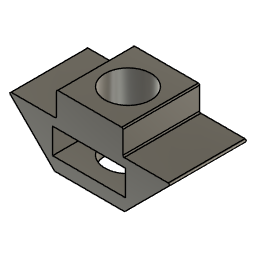
t-slot-nut (Autodesk Fusion 360 design; units mm, degrees)
Autodesk Fusion 360 part; units mm, degrees
sketch "Sketch1" plane through (0, 0, 0) normal (0, 1, 0) x (1, 0, 0) in component "2020-extrusion v1"
  line L0 (9, -10) -> (-9, -10)
  line L1 (-10, -9) -> (-10, 9)
  line L2 (-9, 10) -> (9, 10)
  line L3 (10, 9) -> (10, -9)
  line L4 (10, -10) -> (-10, 10) construction
  line L5 (-10, -10) -> (10, 10) construction
  line L6 (4, -4) -> (-4, -4)
  line L7 (-4, -4) -> (-4, 4)
  line L8 (-4, 4) -> (4, 4)
  line L9 (4, 4) -> (4, -4)
  line L10 (4, -4) -> (-4, 4) construction
  line L11 (-4, -4) -> (4, 4) construction
  circle A0 centre (0, 0) radius 2
  line L12 (8.45, -8.45) -> (-8.45, -8.45)
  line L13 (-8.45, -8.45) -> (-8.45, 8.45)
  line L14 (-8.45, 8.45) -> (8.45, 8.45)
  line L15 (8.45, 8.45) -> (8.45, -8.45)
  line L16 (8.45, -8.45) -> (-8.45, 8.45) construction
  line L17 (-8.45, -8.45) -> (8.45, 8.45) construction
  line L18 (-9.452, -10.548) -> (10.548, 9.452) construction
  line L19 (-10.548, -9.452) -> (9.452, 10.548) construction
  line L20 (10.548, -9.452) -> (-9.452, 10.548) construction
  line L21 (9.452, -10.548) -> (-10.548, 9.452) construction
  line L22 (3.1, -10) -> (-3.1, -10) construction
  line L23 (-3.1, -10) -> (-3.1, 10) construction
  line L24 (-3.1, 10) -> (3.1, 10) construction
  line L25 (3.1, 10) -> (3.1, -10) construction
  line L26 (10, -3.1) -> (-10, -3.1) construction
  line L27 (-10, -3.1) -> (-10, 3.1) construction
  line L28 (-10, 3.1) -> (10, 3.1) construction
  line L29 (10, 3.1) -> (10, -3.1) construction
  line L30 (-3.1, -8.45) -> (-3.1, -10)
  line L31 (3.1, -8.45) -> (3.1, -10)
  line L32 (-8.45, -3.1) -> (-10, -3.1)
  line L33 (-8.45, 3.1) -> (-10, 3.1)
  line L34 (8.45, -3.1) -> (10, -3.1)
  line L35 (8.45, 3.1) -> (10, 3.1)
  line L36 (-3.1, 8.45) -> (-3.1, 10)
  line L37 (3.1, 8.45) -> (3.1, 10)
  line L38 (-4, 2.904) -> (-8.45, 7.354)
  line L39 (-2.904, 4) -> (-7.354, 8.45)
  line L40 (2.904, 4) -> (7.354, 8.45)
  line L41 (4, 2.904) -> (8.45, 7.354)
  line L42 (-4, -2.904) -> (-8.45, -7.354)
  line L43 (-2.904, -4) -> (-7.354, -8.45)
  line L44 (2.904, -4) -> (7.354, -8.45)
  line L45 (4, -2.904) -> (8.45, -7.354)
  line L46 (-10, -3.1) -> (-9.55, -3.1)
  line L47 (-9.55, -3.1) -> (-9.55, -3.6)
  line L48 (-9.55, -3.6) -> (-10, -3.6)
  line L49 (-10, -3.6) -> (-10, -3.1)
  line L50 (-10, 3.1) -> (-9.55, 3.1)
  line L51 (-9.55, 3.1) -> (-9.55, 3.6)
  line L52 (-9.55, 3.6) -> (-10, 3.6)
  line L53 (-10, 3.6) -> (-10, 3.1)
  line L54 (-3.1, -10) -> (-3.6, -10)
  line L55 (-3.6, -10) -> (-3.6, -9.55)
  line L56 (-3.6, -9.55) -> (-3.1, -9.55)
  line L57 (-3.1, -9.55) -> (-3.1, -10)
  line L58 (3.1, -10) -> (3.6, -10)
  line L59 (3.6, -10) -> (3.6, -9.55)
  line L60 (3.6, -9.55) -> (3.1, -9.55)
  line L61 (3.1, -9.55) -> (3.1, -10)
  line L62 (10, -3.1) -> (9.55, -3.1)
  line L63 (9.55, -3.1) -> (9.55, -3.6)
  line L64 (9.55, -3.6) -> (10, -3.6)
  line L65 (10, -3.6) -> (10, -3.1)
  line L66 (10, 3.1) -> (9.55, 3.1)
  line L67 (9.55, 3.1) -> (9.55, 3.6)
  line L68 (9.55, 3.6) -> (10, 3.6)
  line L69 (10, 3.6) -> (10, 3.1)
  line L70 (-3.1, 10) -> (-3.6, 10)
  line L71 (-3.6, 10) -> (-3.6, 9.55)
  line L72 (-3.6, 9.55) -> (-3.1, 9.55)
  line L73 (-3.1, 9.55) -> (-3.1, 10)
  line L74 (3.1, 10) -> (3.55, 10)
  line L75 (3.55, 10) -> (3.55, 9.5)
  line L76 (3.55, 9.5) -> (3.1, 9.5)
  line L77 (3.1, 9.5) -> (3.1, 10)
  arc A1 (-10, -9) -> (-9, -10) centre (-9, -9) ccw
  arc A2 (9, -10) -> (10, -9) centre (9, -9) ccw
  arc A3 (10, 9) -> (9, 10) centre (9, 9) ccw
  arc A4 (-9, 10) -> (-10, 9) centre (-9, 9) ccw
  dimension "d1" = 20
  dimension "d2" = 20
  dimension "d3" = 8
  dimension "d4" = 8
  dimension "d5" = 4
  dimension "d6" = 16.9
  dimension "d7" = 16.9
  dimension "d8" = 0.775
  dimension "d9" = -0.775
  dimension "d10" = 0.775
  dimension "d11" = -0.775
  dimension "d12" = 6.2
  dimension "d13" = 20
  dimension "d14" = 20
  dimension "d15" = 6.2
  dimension "d16" = 1.55
  dimension "d17" = 1.55
  dimension "d18" = 1.55
  dimension "d19" = 1.55
  dimension "d20" = 1.55
  dimension "d21" = 1.55
  dimension "d22" = 1.55
  dimension "d23" = 1.55
  dimension "d24" = 0.45
  dimension "d25" = 0.5
  dimension "d26" = 0.45
  dimension "d27" = 0.5
  dimension "d28" = 0.5
  dimension "d29" = 0.45
  dimension "d30" = 0.5
  dimension "d31" = 0.45
  dimension "d32" = 0.45
  dimension "d33" = 0.5
  dimension "d34" = 0.45
  dimension "d35" = 0.5
  dimension "d36" = 0.5
  dimension "d37" = 0.45
  dimension "d38" = 0.45
  dimension "d39" = 0.5
  dimension "d40" = 1
  dimension "d41" = 1
  dimension "d42" = 1
  dimension "d43" = 1
  constraint horizontal L0
  constraint perpendicular L0 L1
  constraint parallel L0 L2
  constraint parallel L1 L3
  constraint coincident L4 A0.centre
  constraint coincident L5 A0.centre
  constraint coincident A0.centre origin
  constraint horizontal L6
  constraint perpendicular L6 L7
  constraint parallel L6 L8
  constraint parallel L7 L9
  constraint coincident L10 A0.centre
  constraint coincident L11 A0.centre
  constraint horizontal L12
  constraint perpendicular L12 L13
  constraint parallel L12 L14
  constraint parallel L13 L15
  constraint coincident L16 A0.centre
  constraint coincident L17 A0.centre
  constraint horizontal L22
  constraint perpendicular L22 L23
  constraint parallel L22 L24
  constraint parallel L23 L25
  constraint horizontal L26
  constraint perpendicular L26 L27
  constraint parallel L26 L28
  constraint parallel L27 L29
  constraint vertical L30
  constraint coincident L23 L30.start
  constraint coincident L12 L30.start
  constraint vertical L31
  constraint coincident L12 L31.start
  constraint coincident L25 L31.start
  constraint horizontal L32
  constraint coincident L13 L32.start
  constraint coincident L26 L32.start
  constraint horizontal L33
  constraint coincident L13 L33.start
  constraint coincident L28 L33.start
  constraint horizontal L34
  constraint coincident L15 L34.start
  constraint coincident L26 L34.start
  constraint coincident L28 L35.start
  constraint coincident L15 L35.start
  constraint perpendicular L3 L35
  constraint vertical L36
  constraint coincident L14 L36.start
  constraint coincident L23 L36.start
  constraint vertical L37
  constraint coincident L14 L37.start
  constraint coincident L25 L37.start
  constraint coincident L21 L38.start
  constraint coincident L7 L38.start
  constraint coincident L21 L38.end
  constraint coincident L13 L38.end
  constraint coincident L8 L39.start
  constraint coincident L20 L39.start
  constraint coincident L14 L39.end
  constraint coincident L20 L39.end
  constraint coincident L8 L40.start
  constraint coincident L19 L40.start
  constraint coincident L19 L40.end
  constraint coincident L14 L40.end
  constraint coincident L18 L41.start
  constraint coincident L9 L41.start
  constraint coincident L18 L41.end
  constraint coincident L15 L41.end
  constraint coincident L7 L42.start
  constraint coincident L19 L42.start
  constraint coincident L19 L42.end
  constraint coincident L13 L42.end
  constraint coincident L18 L43.start
  constraint coincident L6 L43.start
  constraint coincident L18 L43.end
  constraint coincident L12 L43.end
  constraint coincident L6 L44.start
  constraint coincident L21 L44.start
  constraint coincident L12 L44.end
  constraint coincident L21 L44.end
  constraint coincident L9 L45.start
  constraint coincident L20 L45.start
  constraint coincident L20 L45.end
  constraint coincident L15 L45.end
  constraint horizontal L46
  constraint vertical L47
  constraint horizontal L48
  constraint vertical L49
  constraint horizontal L50
  constraint vertical L51
  constraint horizontal L52
  constraint vertical L53
  constraint horizontal L54
  constraint vertical L55
  constraint horizontal L56
  constraint vertical L57
  constraint horizontal L58
  constraint vertical L59
  constraint horizontal L60
  constraint vertical L61
  constraint horizontal L62
  constraint vertical L63
  constraint horizontal L64
  constraint vertical L65
  constraint horizontal L66
  constraint vertical L67
  constraint horizontal L68
  constraint vertical L69
  constraint horizontal L70
  constraint vertical L71
  constraint horizontal L72
  constraint vertical L73
  constraint horizontal L74
  constraint vertical L75
  constraint horizontal L76
  constraint vertical L77
  constraint coincident L5.start L0
  constraint coincident L5.start L1
  constraint tangent L0 A1
  constraint tangent L1 A1
  constraint coincident L4.start L0
  constraint coincident L4.start L3
  constraint tangent L0 A2
  constraint tangent L3 A2
  constraint coincident L5.end L3
  constraint coincident L5.end L2
  constraint tangent L3 A3
  constraint tangent L2 A3
  constraint coincident L4.end L2
  constraint coincident L4.end L1
  constraint tangent L2 A4
  constraint tangent L1 A4
  measures "d1" distance of L4.end L5.end
  measures "d2" distance of L5.start L4.end
  measures "d3" distance of L7.end L8.end
  measures "d4" distance of L6.end L7.end
  measures "d5" diameter of A0
  measures "d6" distance of L13.end L14.end
  measures "d7" distance of L12.end L13.end
  measures "d12" distance of L23.end L24.end
  measures "d13" distance of L22.end L23.end
  measures "d14" distance of L27.end L28.end
  measures "d15" distance of L26.end L27.end
  measures "d16" distance of L30.start L22.end
  measures "d17" distance of L31.start L22.start
  measures "d18" distance of L32.start L26.end
  measures "d19" distance of L33.start L27.end
  measures "d20" distance of L34.start L26.start
  measures "d21" distance of L35.start L28.end
  measures "d22" distance of L36.start L23.end
  measures "d23" distance of L37.start L24.end
  measures "d24" distance of L26.end L46.end
  measures "d25" distance of L26.end L48.end
  measures "d26" distance of L27.end L50.end
  measures "d27" distance of L27.end L52.end
  measures "d28" distance of L22.end L54.end
  measures "d29" distance of L22.end L56.end
  measures "d30" distance of L22.start L58.end
  measures "d31" distance of L22.start L60.end
  measures "d32" distance of L26.start L62.end
  measures "d33" distance of L26.start L64.end
  measures "d34" distance of L28.end L66.end
  measures "d35" distance of L28.end L68.end
  measures "d36" distance of L23.end L70.end
  measures "d37" distance of L23.end L72.end
  measures "d38" distance of L24.end L74.end
  measures "d39" distance of L24.end L76.end
  measures "d40" radius of A1
  measures "d41" radius of A2
  measures "d42" radius of A3
  measures "d43" radius of A4
extrude "Extrude1" add sketch "Sketch1" along normal blind 500 contours L0 L3 L12 L15 L31 L34 L59 L60 L63 L64 A2 | L0 L1 L12 L13 L30 L32 L47 L48 L55 L56 A1 | L6 L9 L12 L15 L44 L45 | L2 L3 L14 L15 L35 L37 L67 L68 L75 L76 A3 | L6 L7 L12 L13 L42 L43 | L6 L7 L8 L9 | L8 L9 L14 L15 L40 L41 | L1 L2 L13 L14 L33 L36 L51 L52 L71 L72 A4 | L7 L8 L13 L14 L38 L39 makes body 1 in component "2020-extrusion v1"
fillet "Fillet1" radius 0.5 16 edges at (-8.45, 250, -7.354) (-7.354, 250, -8.45) (7.354, 250, -8.45) (8.45, 250, -7.354) (8.45, 250, 7.354) (7.354, 250, 8.45) (-7.354, 250, 8.45) (-8.45, 250, 7.354) (-2.904, 250, 4) (2.904, 250, 4) (-4, 250, 2.904) (-4, 250, -2.904) (-2.904, 250, -4) (2.904, 250, -4) (4, 250, -2.904) (4, 250, 2.904) on bodies 1 in component "2020-extrusion v1"
sketch "Sketch1 (2)" plane through (0, 0, 0) normal (0, -1, 0) x (1, 0, 0)
  circle A0 centre (0, 0) radius 2
  line L0 (-9, -10) -> (-3.6, -10)
  line L1 (-3.6, -10) -> (-3.6, -9.55)
  line L2 (-3.6, -9.55) -> (-3.1, -9.55)
  line L3 (-3.1, -9.55) -> (-3.1, -8.45)
  line L4 (-3.1, -8.45) -> (-6.1469, -8.45)
  arc A1 (-6.5004, -7.5964) -> (-6.1469, -8.45) centre (-6.1469, -7.95) ccw
  line L5 (-6.5004, -7.5964) -> (-3.0504, -4.1464)
  arc A2 (-2.6969, -4) -> (-3.0504, -4.1464) centre (-2.6969, -4.5) ccw
  line L6 (-2.6969, -4) -> (2.6969, -4)
  arc A3 (3.0504, -4.1464) -> (2.6969, -4) centre (2.6969, -4.5) ccw
  line L7 (3.0504, -4.1464) -> (6.5004, -7.5964)
  arc A4 (6.1469, -8.45) -> (6.5004, -7.5964) centre (6.1469, -7.95) ccw
  line L8 (6.1469, -8.45) -> (3.1, -8.45)
  line L9 (3.1, -8.45) -> (3.1, -9.5)
  line L10 (3.1, -9.5) -> (3.55, -9.5)
  line L11 (3.55, -9.5) -> (3.55, -10)
  line L12 (3.55, -10) -> (9, -10)
  arc A5 (9, -10) -> (10, -9) centre (9, -9) ccw
  line L13 (10, -9) -> (10, -3.6)
  line L14 (10, -3.6) -> (9.55, -3.6)
  line L15 (9.55, -3.6) -> (9.55, -3.1)
  line L16 (9.55, -3.1) -> (8.45, -3.1)
  line L17 (8.45, -3.1) -> (8.45, -6.1469)
  arc A6 (7.5964, -6.5004) -> (8.45, -6.1469) centre (7.95, -6.1469) ccw
  line L18 (7.5964, -6.5004) -> (4.1464, -3.0504)
  arc A7 (4, -2.6969) -> (4.1464, -3.0504) centre (4.5, -2.6969) ccw
  line L19 (4, -2.6969) -> (4, 2.6969)
  arc A8 (4.1464, 3.0504) -> (4, 2.6969) centre (4.5, 2.6969) ccw
  line L20 (4.1464, 3.0504) -> (7.5964, 6.5004)
  arc A9 (8.45, 6.1469) -> (7.5964, 6.5004) centre (7.95, 6.1469) ccw
  line L21 (8.45, 6.1469) -> (8.45, 3.1)
  line L22 (8.45, 3.1) -> (9.55, 3.1)
  line L23 (9.55, 3.1) -> (9.55, 3.6)
  line L24 (9.55, 3.6) -> (10, 3.6)
  line L25 (10, 3.6) -> (10, 9)
  arc A10 (10, 9) -> (9, 10) centre (9, 9) ccw
  line L26 (9, 10) -> (3.6, 10)
  line L27 (3.6, 10) -> (3.6, 9.55)
  line L28 (3.6, 9.55) -> (3.1, 9.55)
  line L29 (3.1, 9.55) -> (3.1, 8.45)
  line L30 (3.1, 8.45) -> (6.1469, 8.45)
  arc A11 (6.5004, 7.5964) -> (6.1469, 8.45) centre (6.1469, 7.95) ccw
  line L31 (6.5004, 7.5964) -> (3.0504, 4.1464)
  arc A12 (2.6969, 4) -> (3.0504, 4.1464) centre (2.6969, 4.5) ccw
  line L32 (2.6969, 4) -> (-2.6969, 4)
  arc A13 (-3.0504, 4.1464) -> (-2.6969, 4) centre (-2.6969, 4.5) ccw
  line L33 (-3.0504, 4.1464) -> (-6.5004, 7.5964)
  arc A14 (-6.1469, 8.45) -> (-6.5004, 7.5964) centre (-6.1469, 7.95) ccw
  line L34 (-6.1469, 8.45) -> (-3.1, 8.45)
  line L35 (-3.1, 8.45) -> (-3.1, 9.55)
  line L36 (-3.1, 9.55) -> (-3.6, 9.55)
  line L37 (-3.6, 9.55) -> (-3.6, 10)
  line L38 (-3.6, 10) -> (-9, 10)
  arc A15 (-9, 10) -> (-10, 9) centre (-9, 9) ccw
  line L39 (-10, 9) -> (-10, 3.6)
  line L40 (-10, 3.6) -> (-9.55, 3.6)
  line L41 (-9.55, 3.6) -> (-9.55, 3.1)
  line L42 (-9.55, 3.1) -> (-8.45, 3.1)
  line L43 (-8.45, 3.1) -> (-8.45, 6.1469)
  arc A16 (-7.5964, 6.5004) -> (-8.45, 6.1469) centre (-7.95, 6.1469) ccw
  line L44 (-7.5964, 6.5004) -> (-4.1464, 3.0504)
  arc A17 (-4, 2.6969) -> (-4.1464, 3.0504) centre (-4.5, 2.6969) ccw
  line L45 (-4, 2.6969) -> (-4, -2.6969)
  arc A18 (-4.1464, -3.0504) -> (-4, -2.6969) centre (-4.5, -2.6969) ccw
  line L46 (-4.1464, -3.0504) -> (-7.5964, -6.5004)
  arc A19 (-8.45, -6.1469) -> (-7.5964, -6.5004) centre (-7.95, -6.1469) ccw
  line L47 (-8.45, -6.1469) -> (-8.45, -3.1)
  line L48 (-8.45, -3.1) -> (-9.55, -3.1)
  line L49 (-9.55, -3.1) -> (-9.55, -3.6)
  line L50 (-9.55, -3.6) -> (-10, -3.6)
  line L51 (-10, -3.6) -> (-10, -9)
  arc A20 (-10, -9) -> (-9, -10) centre (-9, -9) ccw
  line L52 (-3.1, 8.45) -> (3.1, 8.45)
  line L53 (-3.1, 8.05) -> (3.1, 8.05)
  line L54 (3.1, 8.05) -> (6.1469, 8.05)
  arc A21 (6.2176, 7.8793) -> (6.1469, 8.05) centre (6.1469, 7.95) ccw
  line L55 (6.2176, 7.8793) -> (2.7676, 4.4293)
  arc A22 (2.6969, 4.4) -> (2.7676, 4.4293) centre (2.6969, 4.5) ccw
  line L56 (2.6969, 4.4) -> (-2.6969, 4.4)
  arc A23 (-2.7676, 4.4293) -> (-2.6969, 4.4) centre (-2.6969, 4.5) ccw
  line L57 (-2.7676, 4.4293) -> (-6.2176, 7.8793)
  arc A24 (-6.1469, 8.05) -> (-6.2176, 7.8793) centre (-6.1469, 7.95) ccw
  line L58 (-6.1469, 8.05) -> (-3.1, 8.05)
  line L59 (-3.1, 8.05) -> (2.802, 8.05) construction
  line L60 (2.802, 8.05) -> (2.802, 4.1083) construction
  line L61 (2.802, 4.1083) -> (-3.1, 4.1083) construction
  line L62 (-3.1, 4.1083) -> (-3.1, 8.05) construction
  line L63 (-3.1, 8.05) -> (2.802, 4.1083) construction
  line L64 (2.802, 8.05) -> (-3.1, 4.1083) construction
  line L65 (2.8, 7.375) -> (-2.9, 7.375)
  line L66 (-2.9, 7.375) -> (-2.9, 5.375)
  line L67 (-2.9, 5.375) -> (2.8, 5.375)
  line L68 (2.8, 5.375) -> (2.8, 7.375)
  line L69 (-0.149, 6.0792) -> (-0.149, 6.2792) construction
  line L70 (-3.1, 8.05) -> (-3.1, 10)
  line L71 (-3.1, 10) -> (3.1, 10)
  line L72 (3.1, 10) -> (3.1, 8.05)
  line L73 (-3.1, 10) -> (3.1, 8.05) construction
  line L74 (3.1, 10) -> (-3.1, 8.05) construction
  line L75 (2.6, 10) -> (-2.6, 10)
  line L76 (-2.6, 10) -> (-2.6, 8.05)
  line L77 (-2.6, 8.05) -> (2.6, 8.05)
  line L78 (2.6, 8.05) -> (2.6, 10)
  line L79 (2.6, 10) -> (-2.6, 8.05) construction
  line L80 (-2.6, 10) -> (2.6, 8.05) construction
  point P0 (-0.149, 6.0792)
  point P1 (0, 9.025)
  dimension "d48" = -0.4
  dimension "d49" = 5.7
  dimension "d50" = 2
  dimension "d58" = 0.2
  dimension "d60" = 0
  dimension "d63" = 5.2
  dimension "d64" = 1.95
  constraint coincident L34.end L35.start
  constraint coincident L29.end L30.start
  constraint horizontal L59
  constraint vertical L60
  constraint horizontal L61
  constraint vertical L62
  constraint horizontal L65
  constraint perpendicular L65 L66
  constraint parallel L65 L67
  constraint parallel L66 L68
  constraint midpoint L63 P0
  constraint coincident P0 L69.start
  constraint vertical L69
  constraint perpendicular L38 L70
  constraint perpendicular L29 L71
  constraint perpendicular L54 L72
  constraint horizontal L75
  constraint perpendicular L75 L76
  constraint parallel L75 L77
  constraint parallel L76 L78
  constraint coincident L79 P1
  constraint coincident L80 P1
  constraint midpoint L73 P1
  measures "d49" distance of L66.end L67.end
  measures "d50" distance of L65.end L66.end
  measures "d58" distance of P0 L69.end
  measures "d63" distance of L76.end L77.end
  measures "d64" distance of L75.end L76.end
extrude "Extrude1'" add sketch "Sketch1 (2)" along normal blind 6 separate body contours L53 L54 A21 L55 A22 L56 A23 L57 A24 L58 L77 makes body 2
extrude "Extrude3" add sketch "Sketch1 (2)" along normal blind 0.6 contours L65 L66 L67 L68 bodies 2
extrude "Extrude6" add sketch "Sketch1 (2)" along normal blind 6 contours L52 L71 L75 L76 L78 | L52 L53 L76 L77 L78 bodies 2
fillet "Fillet1'" radius 0.1 4 edges at (-2.6, -3, 8.05) (-2.6, -3, 10) (2.6, -3, 8.05) (2.6, -3, 10) on bodies 2
sketch "Sketch3" plane through (0, 0, 10) normal (0, 0, 1) x (-1, 0, 0)
  line L0 (-2.5, 6) -> (-2.5, 0)
  line L1 (-2.5, 0) -> (2.5, 0)
  line L2 (2.5, 0) -> (2.5, 6)
  line L3 (2.5, 6) -> (-2.5, 6)
  line L4 (-2.5, 0) -> (2.5, 6) construction
  line L5 (-2.5, 6) -> (2.5, 0) construction
  circle A0 centre (0, 3) radius 1.8
  dimension "d69" = 3.6
  constraint coincident L0.end L1.start
  constraint coincident L2.end L3.start
  constraint coincident L0.start L3.end
  constraint coincident L1.end L2.start
  constraint midpoint L5 A0.centre
  measures "d69" diameter of A0
extrude "Extrude7" cut sketch "Sketch3" against normal blind 5.6 contours A0 bodies 2
component "2020-extrusion v1" placed x (1, 0, 0) y (0, 1, 0) z (0, 0, 1) at (0, 0, 0)
equation "d6 = 20 mm - ( ( 1.55 * 2 ) * 1 mm )"
equation "d7 = 20 mm - ( ( 1.55 * 2 ) * 1 mm )"
equation "d8 = ( 1.55 / 2 ) * 1 mm"
equation "d9 = ( -1.55 / 2 ) * 1 mm"
equation "d10 = ( 1.55 / 2 ) * 1 mm"
equation "d11 = ( -1.55 / 2 ) * 1 mm"
named bodies: "2020-extrusion"
